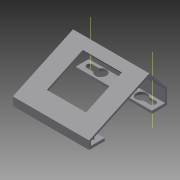
# Autodesk Inventor part: DisplayMount
Saved by Autodesk Inventor 2015 (Build 190159000, 159)
## iProperties
Created: 2022-04-16
Part Number: DisplayMount
Material: Generic
Document SubType Name: Modeling
Designer: Jan
Density: 1 g/cm^3
Appearance: Default
Author: Jan
Autodesk Inventor part; units mm, degrees
ref_plane "XZ Plane" through (0, 0, 0) normal (0, 1, 0) x (-1, 0, 0)
ref_plane "XY Plane" through (0, 0, 0) normal (0, 0, 1) x (1, 0, 0)
sketch "Sketch1" plane through (0, 0, 0) normal (1, 0, 0) x (0, 1, 0)
  line L0 (0, 4.9645) -> (36.2523, 21.8692)
  line L1 (36.2523, 21.8692) -> (47, 9.0606)
  line L2 (45.8, 1.6) -> (45.8, 8.6239)
  line L3 (45.8, 8.6239) -> (35.9249, 20.3925)
  line L4 (35.9249, 20.3925) -> (1.2, 4.2)
  line L5 (0, 4.9645) -> (0, 0)
  line L6 (47, 9.0606) -> (47, 0)
  line L7 (0, 0) -> (9.3, 0)
  line L8 (9.3, 0) -> (9.3, 1.6)
  line L9 (9.3, 1.6) -> (4.8, 1.6)
  line L10 (1.2, 4.2) -> (1.2, 1.6)
  line L11 (45.8, 1.6) -> (42.3, 1.6)
  line L12 (37.8, 1.6) -> (37.8, 0)
  line L13 (37.8, 0) -> (47, 0)
  line L14 (4.8, 1.6) -> (4.8, 0) construction
  line L15 (42.3, 1.6) -> (42.3, 0) construction
  line L16 (42.3, 1.6) -> (37.8, 1.6)
  line L17 (4.8, 1.6) -> (1.2, 1.6)
  dimension "d1" = 1.2
  dimension "d3" = 1.2
  dimension "d4" = 1.2
  dimension "d25" = 40
  dimension "d26" = 25
  dimension "d27" = 1.6
  dimension "d28" = 1.2
  dimension "d29" = 37.5
  dimension "d37" = 105
  dimension "d38" = 4.5
  dimension "d39" = 2.6
  dimension "d42" = 3.5
  dimension "d43" = 3.6
  constraints: 36 end point, 9 perpendicular, 6 collinear, 3 parallel, 3 vertical, 2 horizontal, 2 point on line, 1 coincident
  measures "d1" distance between parallel lines of L2 L6
  measures "d3" distance between parallel lines of L4 L0
  measures "d4" distance between parallel lines of L1 L3
  measures "d25" distance of L0.start L0.end
  measures "d26" angle of L0 L7
  measures "d27" distance between parallel lines of L7 L9
  measures "d28" distance between parallel lines of L10 L5
  measures "d29" distance between parallel lines of L15 L14
  measures "d37" angle of L4 L3
  measures "d38" distance of L11.end L12.start
  measures "d39" distance of L4.end L10.end
  measures "d42" distance of L2.start L11.end
  measures "d43" distance of L9.end L10.end
extrude "Extrusion1" add sketch "Sketch1" along normal mid plane 46
sketch "Sketch3" plane through (23, 35.9249, 20.3925) normal (0, 0.4226, -0.9063) x (-1, 0, 0)
  circle A0 centre (3.405, -5.0219) radius 1.05
  circle A1 centre (37.695, -5.0219) radius 1.05
  circle A2 centre (37.695, -27.9329) radius 1.05
  circle A3 centre (3.405, -27.9329) radius 1.05
  line L0 (0, -39.4135) -> (0, 0) construction
  line L1 (46, 0) -> (46, -39.4135) construction
  circle A4 centre (3.405, -5.0219) radius 1.85
  circle A5 centre (37.695, -5.0219) radius 1.85
  circle A6 centre (37.695, -27.9329) radius 1.85
  circle A7 centre (3.405, -27.9329) radius 1.85
  line L2 (11.205, -4.9754) -> (34.795, -4.9754)
  line L3 (34.795, -4.9754) -> (34.795, -28.7754)
  line L4 (34.795, -28.7754) -> (11.205, -28.7754)
  line L5 (11.205, -28.7754) -> (11.205, -4.9754)
  line L6 (23, -4.9754) -> (23, -28.7754) construction
  line L7 (11.205, -16.8754) -> (0, -16.8754) construction
  line L8 (34.795, -16.8754) -> (46, -16.8754) construction
  point P0 (23, -41.1773)
  dimension "d13" = 34.29
  dimension "d14" = 22.911
  dimension "d15" = 2.1
  dimension "d16" = 0.8
  dimension "d17" = 7.8
  dimension "d18" = 2.9
  dimension "d19" = 23.8
  dimension "d44" = 0.0465
  constraints: 14 end point, 8 centre point, 6 equal radius, 4 coincident, 4 midpoint, 3 perpendicular, 2 horizontal alignment, 2 parallel, 2 point on line, 2 vertical alignment, 1 collinear, 1 horizontal
  measures "d13" distance of A1.centre A0.centre
  measures "d14" distance of A3.centre A0.centre
  measures "d15" diameter of A0
  measures "d16" radial gap between concentric circles of A4 A0
  measures "d17" distance from line of L5 A0.centre
  measures "d18" distance from line of A1.centre L3
  measures "d19" distance between parallel lines of L4 L2
  measures "d44" distance from line of A0.centre L2
extrude "Extrusion2" add sketch "Sketch3" along normal blind 1.7 contours A4 | A5 | A6 | A7
extrude "Extrusion3" cut sketch "Sketch3" against normal up to surface (1.2 mm away) contours L2 L3 L4 L5
sketch "Sketch5" plane through (-23, 0, 0) normal (0, 0, -1) x (-1, 0, 0)
  arc A0 (-4, 3) -> (-4, 6.6) centre (-4, 4.8) ccw
  arc A1 (-42, 6.6) -> (-42, 3) centre (-42, 4.8) ccw
  arc A2 (-42, 44.1) -> (-42, 40.5) centre (-42, 42.3) ccw
  arc A3 (-4, 40.5) -> (-4, 44.1) centre (-4, 42.3) ccw
  line L0 (0, 9.3) -> (0, 0) construction
  line L1 (-46, 9.3) -> (0, 9.3) construction
  line L2 (-46, 0) -> (-46, 9.3) construction
  line L3 (-46, 0) -> (0, 0) construction
  line L4 (0, 47) -> (0, 37.8) construction
  line L5 (-46, 47) -> (0, 47) construction
  line L6 (-46, 37.8) -> (-46, 47) construction
  line L7 (-46, 37.8) -> (0, 37.8) construction
  line L8 (-23, -9.4) -> (-23, 56.4) projected
  arc A4 (-8, 6.6) -> (-8, 3) centre (-8, 4.8) ccw construction
  line L9 (-4, 6.6) -> (-8, 6.6)
  line L10 (-4, 3) -> (-8, 3)
  arc A5 (-38, 3) -> (-38, 6.6) centre (-38, 4.8) ccw construction
  arc A6 (-38, 40.5) -> (-38, 44.1) centre (-38, 42.3) ccw construction
  arc A7 (-8, 44.1) -> (-8, 40.5) centre (-8, 42.3) ccw construction
  line L11 (-38, 3) -> (-42, 3)
  line L12 (-38, 6.6) -> (-42, 6.6)
  line L13 (-38, 40.5) -> (-42, 40.5)
  line L14 (-42, 44.1) -> (-38, 44.1)
  line L15 (-4, 44.1) -> (-8, 44.1)
  line L16 (-8, 40.5) -> (-4, 40.5)
  arc A8 (-8, 6.6) -> (-8, 3) centre (-10.7659, 4.8) ccw
  arc A9 (-38, 3) -> (-38, 6.6) centre (-35.2341, 4.8) ccw
  arc A10 (-8, 44.1) -> (-8, 40.5) centre (-10.7659, 42.3) ccw
  arc A11 (-38, 40.5) -> (-38, 44.1) centre (-35.2341, 42.3) ccw
  point P0 (-23, 0)
  point P1 (-23, 4.8)
  dimension "d30" = 37.5
  dimension "d31" = 38
  dimension "d32" = 3.6
  dimension "d33" = 4
  dimension "d34" = 6.6
  constraints: 24 point on circle, 18 end point, 16 tangent, 12 centre point, 8 horizontal, 7 horizontal alignment, 6 equal radius, 4 vertical alignment, 2 symmetric about line
  measures "d30" distance of A3.centre A0.centre
  measures "d31" distance of A1.centre A0.centre
  measures "d32" diameter of A0
  measures "d33" distance of A4.centre A0.centre
  measures "d34" diameter of A8
extrude "Extrusion4" cut sketch "Sketch5" against normal up to next
ref_plane "Work Plane1" through (18.75, 0, 0) normal (1, 0, 0) x (0, 1, 0)
ref_plane "Work Plane2" through (-18.75, 0, 0) normal (1, 0, 0) x (0, 1, 0)
ref_plane "Work Plane3" through (15, 42.3, 1.6) normal (0, -1, 0) x (1, 0, 0)
body "Solid1"
